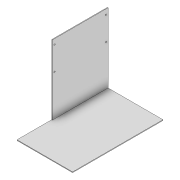
# Autodesk Inventor part: df
Saved by Autodesk Inventor 2021 (Build 250183000, 183)
## iProperties
Created: 2021-06-28
Part Number: df
Material: Generic
Document SubType Name: Modeling
Designer: Shaheen Khan
Density: 1 g/cm^3
Appearance: Default
Author: Shaheen Khan
Autodesk Inventor part; units mm, degrees
ref_plane "YZ Plane" through (0, 0, 0) normal (1, 0, 0) x (0, 1, 0)
ref_plane "XZ Plane" through (0, 0, 0) normal (0, 1, 0) x (-1, 0, 0)
ref_plane "XY Plane" through (0, 0, 0) normal (0, 0, 1) x (1, 0, 0)
sketch "Sketch1" plane through (0, 0, 0) normal (0, 1, 0) x (-1, 0, 0)
  line L0 (-200, 325) -> (200, 325)
  line L1 (200, 325) -> (200, -325)
  line L2 (200, -325) -> (-200, -325)
  line L3 (-200, -325) -> (-200, 325)
  line L4 (-200, 325) -> (200, -325) construction
  line L5 (200, 325) -> (-200, -325) construction
  point P0 (0, 0)
  dimension "d0" = 650
  dimension "d1" = 400
  constraints: 12 end point, 2 midpoint, 2 parallel, 1 horizontal, 1 perpendicular
  measures "d0" distance of L0.end L1.end
  measures "d1" distance of L0.start L0.end
extrude "Extrusion1" add sketch "Sketch1" along normal blind 5
sketch "Sketch2" plane through (200, 0, -325) normal (0, 0, -1) x (-1, 0, 0)
  line L0 (0, 5) -> (400, 5) projected
  line L1 (400, 5) -> (395, 5)
  line L2 (395, 5) -> (395, 505)
  line L3 (395, 505) -> (400, 505)
  line L4 (400, 505) -> (400, 5)
  point P0 (200, 0)
  dimension "d4" = 5
  dimension "d5" = 500
  constraints: 8 end point, 2 parallel, 1 horizontal, 1 perpendicular
  measures "d4" distance of L2.end L3.end
  measures "d5" distance of L1.end L2.end
extrude "Extrusion2" add sketch "Sketch2" against normal blind 400
sketch "Sketch3" plane through (-195, 5, -325) normal (1, 0, 0) x (0, 0, -1)
  line L0 (-400, 0) -> (-400, 500) projected
  line L1 (0, 500) -> (0, 0) projected
  point P0 (-325, -5)
  point P1 (-385, 463.2751)
  point P2 (-15, 463.2751)
  point P3 (-15, 293.2751)
  point P4 (-385, 293.2751)
  dimension "d8" = 15
  dimension "d9" = 15
  dimension "d10" = 170
  constraints: 2 horizontal alignment, 2 vertical alignment
  measures "d8" distance from line of point (-385, 463.275) L0
  measures "d9" distance from line of L1 point (-15, 463.275)
  measures "d10" distance of point (-385, 293.275) point (-385, 463.275)
hole "Hole1" at (-195, 468.2751, 60) at (-195, 468.2751, -310) at (-195, 298.2751, -310) at (-195, 298.2751, 60) direction (-1, 0, 0) diameter 10 end through all
body "Solid1"
